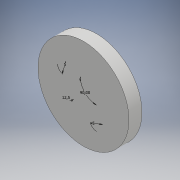
# Autodesk Inventor part: Part11
Saved by Autodesk Inventor 2017 (Build 210142000, 142)
## iProperties
Created: 2021-05-19
Part Number: Part11
Material: Generic
Document SubType Name: Modeling
Designer: majch
Density: 1 g/cm^3
Appearance: Default
Author: majch
Autodesk Inventor part; units mm, degrees
ref_plane "YZ Plane" through (0, 0, 0) normal (1, 0, 0) x (0, 1, 0)
ref_plane "XZ Plane" through (0, 0, 0) normal (0, 1, 0) x (-1, 0, 0)
ref_plane "XY Plane" through (0, 0, 0) normal (0, 0, 1) x (1, 0, 0)
sketch "Sketch1" plane through (0, 0, 0) normal (0, 1, 0) x (-1, 0, 0)
  circle A0 centre (0, 0) radius 17.5
  dimension "d0" = 35
  constraints: 1 centre point, 1 coincident
  measures "d0" diameter of A0
extrude "Extrusion1" add sketch "Sketch1" along normal blind 5
sketch "Sketch2" plane through (0, 5, 0) normal (0, 1, 0) x (1, 0, 0)
  arc A0 (0, 12.5) -> (-12.5, 0) centre (0, 0) ccw construction
  line L0 (0, 0) -> (0, 12.5) construction
  line L1 (0, 0) -> (-12.5, 0) construction
  arc A1 (-15, 0) -> (-10, 0) centre (-12.5, 0) ccw
  arc A2 (0, 10) -> (0, 15) centre (0, 12.5) ccw
  arc A3 (0, 10) -> (-10, 0) centre (0, 0) ccw
  arc A4 (0, 15) -> (-15, 0) centre (0, 0) ccw
  dimension "d4" = 12.5
  dimension "kat" = 90
  dimension "d6" = 5
  dimension "d7" = 5
  constraints: 10 point on circle, 7 coincident, 5 centre point, 4 end point, 2 point on line
  measures "d4" radius of A0
  measures "kat" angle of L0 L1
  measures "d6" diameter of A1
  measures "d7" diameter of A2
body "Solid1"
